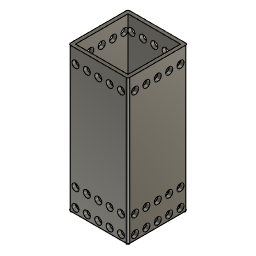
airbee_base (Autodesk Fusion 360 design; units mm, degrees)
Autodesk Fusion 360 part; units mm, degrees
sketch "Skizze1" plane through (0, 0, 0) normal (0, 0, 1) x (1, 0, 0)
  line L0 (-15, 15) -> (15, 15)
  line L1 (15, 15) -> (15, -15)
  line L2 (15, -15) -> (-15, -15)
  line L3 (-15, -15) -> (-15, 15)
  line L4 (17, -17) -> (-17, -17)
  line L5 (-17, -17) -> (-17, 17)
  line L6 (-17, 17) -> (17, 17)
  line L7 (17, 17) -> (17, -17)
  circle A0 centre (-10.16, 6.35) radius 3.5
  circle A1 centre (10.16, 6.35) radius 3.5
  circle A2 centre (-10.16, -6.35) radius 3.5
  circle A3 centre (10.16, -6.35) radius 3.5
  circle A4 centre (-10.16, 6.35) radius 0.75
  circle A5 centre (10.16, 6.35) radius 0.75
  circle A6 centre (10.16, -6.35) radius 0.75
  circle A7 centre (-10.16, -6.35) radius 0.75
  line L8 (-15, 3.5) -> (15, 3.5)
  line L9 (15, 3.5) -> (15, -3.5)
  line L10 (15, -3.5) -> (-15, -3.5)
  line L11 (-15, -3.5) -> (-15, 3.5)
  dimension "d3" = 30
  dimension "d4" = 30
  dimension "d5" = 15
  dimension "d6" = 15
  dimension "d7" = -2
  dimension "d8" = 7
  dimension "d9" = 7
  dimension "d10" = 7
  dimension "d11" = 7
  dimension "d12" = 20.32
  dimension "d16" = 4.84
  dimension "d19" = 4.84
  dimension "d20" = 12.7
  dimension "d21" = 20.32
  dimension "d22" = 12.7
  dimension "d23" = 8.65
  dimension "d25" = 8.65
  dimension "d26" = 1.5
  dimension "d27" = 1.5
  dimension "d28" = 1.5
  dimension "d29" = 1.5
  dimension "d140" = 7
  dimension "d141" = 3.5
  constraint horizontal L0
  constraint vertical L1
  constraint horizontal L2
  constraint vertical L3
  constraint concentric A0 A4
  constraint concentric A1 A5
  constraint concentric A3 A6
  constraint concentric A2 A7
  constraint horizontal L8
  constraint vertical L9
  constraint horizontal L10
  constraint vertical L11
  constraint coincident L1 L9.end
  constraint coincident L3 L8.start
  measures "d3" distance of L0.start L0.end
  measures "d4" distance of L0.start L2.end
  measures "d5" distance of origin L1
  measures "d6" distance of origin L2
  measures "d8" diameter of A0
  measures "d9" diameter of A1
  measures "d10" diameter of A3
  measures "d11" diameter of A2
  measures "d12" horizontal distance of A0.centre A1.centre
  measures "d16" distance of L3 A0.centre
  measures "d19" distance of L1 A3.centre
  measures "d20" distance of A1.centre A3.centre
  measures "d21" distance of A2.centre A3.centre
  measures "d22" vertical distance of A0.centre A2.centre
  measures "d23" distance of L0 A0.centre
  measures "d25" distance of L0 A1.centre
  measures "d26" diameter of A4
  measures "d27" diameter of A5
  measures "d28" diameter of A6
  measures "d29" diameter of A7
  measures "d140" distance of L8 L10
  measures "d141" distance of origin L8
extrude "Extrusion1" add sketch "Skizze1" against normal blind 2 contours L0 L1 L3 A0 A1 L8 | L1 L3 A0 A1 A2 A3 L8 L9 L10 L11 | L1 L2 L3 A2 A3 L10 | A0 L8 | A0 L8 | A1 L8 | A1 L8 | A2 L10 | A2 L10 | A3 L10 | A3 L10 | L4 L5 L6 L7 | A4 | A5 | A6 | A7
extrude "Extrusion2" add sketch "Skizze1" along normal blind 81 contours L4 L5 L6 L7
sketch "Skizze10" plane through (17, 0, 0) normal (1, 0, 0) x (0, 1, 0)
  line L0 (-15, 0) -> (15, 0)
  circle A0 centre (13, 2) radius 2
  circle A1 centre (6.5, 2) radius 2
  circle A2 centre (0, 2) radius 2
  circle A3 centre (-6.5, 2) radius 2
  circle A4 centre (-13, 2) radius 2
  circle A5 centre (13, 12.1429) radius 2
  circle A6 centre (6.5, 12.1429) radius 2
  circle A7 centre (0, 12.1429) radius 2
  circle A8 centre (-6.5, 12.1429) radius 2
  circle A9 centre (-13, 12.1429) radius 2
  circle A10 centre (13, 22.2857) radius 2
  circle A11 centre (6.5, 22.2857) radius 2
  circle A12 centre (0, 22.2857) radius 2
  circle A13 centre (-6.5, 22.2857) radius 2
  circle A14 centre (-13, 22.2857) radius 2
  circle A15 centre (13, 32.4286) radius 2
  circle A16 centre (6.5, 32.4286) radius 2
  circle A17 centre (0, 32.4286) radius 2
  circle A18 centre (-6.5, 32.4286) radius 2
  circle A19 centre (-13, 32.4286) radius 2
  circle A20 centre (13, 42.5714) radius 2
  circle A21 centre (6.5, 42.5714) radius 2
  circle A22 centre (0, 42.5714) radius 2
  circle A23 centre (-6.5, 42.5714) radius 2
  circle A24 centre (-13, 42.5714) radius 2
  circle A25 centre (13, 52.7143) radius 2
  circle A26 centre (6.5, 52.7143) radius 2
  circle A27 centre (0, 52.7143) radius 2
  circle A28 centre (-6.5, 52.7143) radius 2
  circle A29 centre (-13, 52.7143) radius 2
  circle A30 centre (13, 62.8571) radius 2
  circle A31 centre (6.5, 62.8571) radius 2
  circle A32 centre (0, 62.8571) radius 2
  circle A33 centre (-6.5, 62.8571) radius 2
  circle A34 centre (-13, 62.8571) radius 2
  circle A35 centre (13, 73) radius 2
  circle A36 centre (6.5, 73) radius 2
  circle A37 centre (0, 73) radius 2
  circle A38 centre (-6.5, 73) radius 2
  circle A39 centre (-13, 73) radius 2
  line L1 (-17, 81) -> (-17, -2)
  line L2 (-17, -2) -> (17, -2)
  line L3 (17, -2) -> (17, 81)
  line L4 (17, 81) -> (-17, 81)
  line L5 (15, 10) -> (-15, 10)
  line L6 (-15, 10) -> (-15, 81)
  line L7 (-15, 81) -> (15, 81)
  line L8 (15, 81) -> (15, 10)
  line L9 (15, 10) -> (-15, 10)
  line L10 (-15, 10) -> (-15, 6)
  line L11 (-15, 6) -> (15, 6)
  line L12 (15, 6) -> (15, 10)
  line L13 (15, 0) -> (15, 81)
  dimension "d146" = 4
  dimension "d151" = -26
  dimension "d152" = 71
  dimension "d197" = 2
  dimension "d198" = 2
  dimension "d199" = 71
  dimension "d200" = 4
  dimension "d201" = 2
  dimension "d202" = 2
  constraint horizontal L5
  constraint vertical L6
  constraint horizontal L7
  constraint vertical L8
  constraint coincident L4 L6.end
  constraint horizontal L9
  constraint vertical L10
  constraint horizontal L11
  constraint vertical L12
  measures "d146" diameter of A0
  measures "d197" distance of L3 L8
  measures "d198" distance of L1 L6
  measures "d199" distance of L5 L7
  measures "d200" distance of L5.start L11.end
  measures "d201" distance of L0 A0.centre
  measures "d202" distance of A0.centre L13
sketch "Skizze16" plane through (0, 17, 0) normal (0, 1, 0) x (-1, 0, 0)
  line L0 (-17, 81) -> (-17, -2)
  line L1 (-17, -2) -> (17, -2)
  line L2 (17, -2) -> (17, 81)
  line L3 (17, 81) -> (-17, 81)
  line L4 (-17, 81) -> (-17, -2)
  circle A0 centre (0, 52.7143) radius 2
  circle A1 centre (-6.5, 22.2857) radius 2
  circle A2 centre (13, 62.8571) radius 2
  circle A3 centre (6.5, 52.7143) radius 2
  line L5 (15, 6) -> (15, 10)
  circle A4 centre (0, 62.8571) radius 2
  circle A5 centre (6.5, 42.5714) radius 2
  circle A6 centre (-6.5, 62.8571) radius 2
  line L6 (-15, 0) -> (15, 0)
  circle A7 centre (13, 42.5714) radius 2
  circle A8 centre (13, 22.2857) radius 2
  circle A9 centre (-6.5, 2) radius 2
  circle A10 centre (6.5, 2) radius 2
  circle A11 centre (-6.5, 73) radius 2
  circle A12 centre (-13, 2) radius 2
  circle A13 centre (13, 73) radius 2
  circle A14 centre (6.5, 73) radius 2
  circle A15 centre (-13, 42.5714) radius 2
  circle A16 centre (13, 2) radius 2
  circle A17 centre (-6.5, 42.5714) radius 2
  line L7 (15, 0) -> (15, 81)
  circle A18 centre (-6.5, 52.7143) radius 2
  circle A19 centre (6.5, 32.4286) radius 2
  circle A20 centre (6.5, 62.8571) radius 2
  circle A21 centre (6.5, 12.1429) radius 2
  circle A22 centre (13, 52.7143) radius 2
  line L8 (15, 10) -> (-15, 10)
  circle A23 centre (-13, 12.1429) radius 2
  circle A24 centre (0, 2) radius 2
  circle A25 centre (-6.5, 12.1429) radius 2
  circle A26 centre (-13, 73) radius 2
  line L9 (-15, 81) -> (15, 81)
  line L10 (17, 81) -> (-17, 81)
  line L11 (-17, -2) -> (17, -2)
  circle A27 centre (13, 12.1429) radius 2
  circle A28 centre (0, 73) radius 2
  circle A29 centre (0, 12.1429) radius 2
  line L12 (-15, 6) -> (15, 6)
  circle A30 centre (13, 32.4286) radius 2
  line L13 (15, 10) -> (-15, 10)
  line L14 (-15, 10) -> (-15, 6)
  circle A31 centre (-6.5, 32.4286) radius 2
  circle A32 centre (-13, 62.8571) radius 2
  circle A33 centre (0, 22.2857) radius 2
  circle A34 centre (6.5, 22.2857) radius 2
  circle A35 centre (-13, 22.2857) radius 2
  circle A36 centre (0, 32.4286) radius 2
  circle A37 centre (-13, 32.4286) radius 2
  circle A38 centre (-13, 52.7143) radius 2
  line L15 (15, 81) -> (15, 10)
  line L16 (17, -2) -> (17, 81)
  line L17 (-15, 10) -> (-15, 81)
  circle A39 centre (0, 42.5714) radius 2
  dimension "d205" = -26
  dimension "d206" = 71
  dimension "d207" = 4
  dimension "d208" = 2
  dimension "d209" = 2
  dimension "d210" = 71
  dimension "d211" = 4
  dimension "d212" = 2
  dimension "d213" = 2
  constraint horizontal L13
  constraint vertical L17
  constraint horizontal L9
  constraint vertical L15
  constraint coincident L9.start L10
  constraint horizontal L8
  constraint vertical L14
  constraint horizontal L12
  constraint vertical L5
  measures "d207" diameter of A16
  measures "d208" distance of L15 L16
  measures "d209" distance of L4 L17
  measures "d210" distance of L9 L13
  measures "d211" distance of L5.start L5.end
  measures "d212" distance of A16.centre L6
  measures "d213" distance of A16.centre L7
sketch "Skizze17" plane through (-17, 0, 0) normal (-1, 0, 0) x (0, -1, 0)
  line L0 (-17, 81) -> (-17, -2)
  line L1 (-17, -2) -> (17, -2)
  line L2 (17, -2) -> (17, 81)
  line L3 (17, 81) -> (-17, 81)
  line L4 (-17, 81) -> (-17, -2)
  circle A0 centre (0, 52.7143) radius 2
  circle A1 centre (-6.5, 22.2857) radius 2
  circle A2 centre (13, 62.8571) radius 2
  circle A3 centre (6.5, 52.7143) radius 2
  line L5 (15, 6) -> (15, 10)
  circle A4 centre (0, 62.8571) radius 2
  circle A5 centre (6.5, 42.5714) radius 2
  circle A6 centre (-6.5, 62.8571) radius 2
  line L6 (-15, 0) -> (15, 0)
  circle A7 centre (13, 42.5714) radius 2
  circle A8 centre (13, 22.2857) radius 2
  circle A9 centre (-6.5, 2) radius 2
  circle A10 centre (6.5, 2) radius 2
  circle A11 centre (-6.5, 73) radius 2
  circle A12 centre (-13, 2) radius 2
  circle A13 centre (13, 73) radius 2
  circle A14 centre (6.5, 73) radius 2
  circle A15 centre (-13, 42.5714) radius 2
  circle A16 centre (13, 2) radius 2
  circle A17 centre (-6.5, 42.5714) radius 2
  line L7 (15, 0) -> (15, 81)
  circle A18 centre (-6.5, 52.7143) radius 2
  circle A19 centre (6.5, 32.4286) radius 2
  circle A20 centre (6.5, 62.8571) radius 2
  circle A21 centre (6.5, 12.1429) radius 2
  circle A22 centre (13, 52.7143) radius 2
  line L8 (15, 10) -> (-15, 10)
  circle A23 centre (-13, 12.1429) radius 2
  circle A24 centre (0, 2) radius 2
  circle A25 centre (-6.5, 12.1429) radius 2
  circle A26 centre (-13, 73) radius 2
  line L9 (-15, 81) -> (15, 81)
  line L10 (17, 81) -> (-17, 81)
  line L11 (-17, -2) -> (17, -2)
  circle A27 centre (13, 12.1429) radius 2
  circle A28 centre (0, 73) radius 2
  circle A29 centre (0, 12.1429) radius 2
  line L12 (-15, 6) -> (15, 6)
  circle A30 centre (13, 32.4286) radius 2
  line L13 (15, 10) -> (-15, 10)
  line L14 (-15, 10) -> (-15, 6)
  circle A31 centre (-6.5, 32.4286) radius 2
  circle A32 centre (-13, 62.8571) radius 2
  circle A33 centre (0, 22.2857) radius 2
  circle A34 centre (6.5, 22.2857) radius 2
  circle A35 centre (-13, 22.2857) radius 2
  circle A36 centre (0, 32.4286) radius 2
  circle A37 centre (-13, 32.4286) radius 2
  circle A38 centre (-13, 52.7143) radius 2
  line L15 (15, 81) -> (15, 10)
  line L16 (17, -2) -> (17, 81)
  line L17 (-15, 10) -> (-15, 81)
  circle A39 centre (0, 42.5714) radius 2
  dimension "d216" = -26
  dimension "d217" = 71
  dimension "d218" = 4
  dimension "d219" = 2
  dimension "d220" = 2
  dimension "d221" = 71
  dimension "d222" = 4
  dimension "d223" = 2
  dimension "d224" = 2
  constraint horizontal L13
  constraint vertical L17
  constraint horizontal L9
  constraint vertical L15
  constraint coincident L9.start L10
  constraint horizontal L8
  constraint vertical L14
  constraint horizontal L12
  constraint vertical L5
  measures "d218" diameter of A16
  measures "d219" distance of L15 L16
  measures "d220" distance of L4 L17
  measures "d221" distance of L9 L13
  measures "d222" distance of L5.start L5.end
  measures "d223" distance of A16.centre L6
  measures "d224" distance of A16.centre L7
sketch "Skizze18" plane through (0, -17, 0) normal (0, -1, 0) x (1, 0, 0)
  line L0 (-17, 81) -> (-17, -2)
  line L1 (-17, -2) -> (17, -2)
  line L2 (17, -2) -> (17, 81)
  line L3 (17, 81) -> (-17, 81)
  line L4 (-17, 81) -> (-17, -2)
  circle A0 centre (0, 52.7143) radius 2
  circle A1 centre (-6.5, 22.2857) radius 2
  circle A2 centre (13, 62.8571) radius 2
  circle A3 centre (6.5, 52.7143) radius 2
  line L5 (15, 6) -> (15, 10)
  circle A4 centre (0, 62.8571) radius 2
  circle A5 centre (6.5, 42.5714) radius 2
  circle A6 centre (-6.5, 62.8571) radius 2
  line L6 (-15, 0) -> (15, 0)
  circle A7 centre (13, 42.5714) radius 2
  circle A8 centre (13, 22.2857) radius 2
  circle A9 centre (-6.5, 2) radius 2
  circle A10 centre (6.5, 2) radius 2
  circle A11 centre (-6.5, 73) radius 2
  circle A12 centre (-13, 2) radius 2
  circle A13 centre (13, 73) radius 2
  circle A14 centre (6.5, 73) radius 2
  circle A15 centre (-13, 42.5714) radius 2
  circle A16 centre (13, 2) radius 2
  circle A17 centre (-6.5, 42.5714) radius 2
  line L7 (15, 0) -> (15, 81)
  circle A18 centre (-6.5, 52.7143) radius 2
  circle A19 centre (6.5, 32.4286) radius 2
  circle A20 centre (6.5, 62.8571) radius 2
  circle A21 centre (6.5, 12.1429) radius 2
  circle A22 centre (13, 52.7143) radius 2
  line L8 (15, 10) -> (-15, 10)
  circle A23 centre (-13, 12.1429) radius 2
  circle A24 centre (0, 2) radius 2
  circle A25 centre (-6.5, 12.1429) radius 2
  circle A26 centre (-13, 73) radius 2
  line L9 (-15, 81) -> (15, 81)
  line L10 (17, 81) -> (-17, 81)
  line L11 (-17, -2) -> (17, -2)
  circle A27 centre (13, 12.1429) radius 2
  circle A28 centre (0, 73) radius 2
  circle A29 centre (0, 12.1429) radius 2
  line L12 (-15, 6) -> (15, 6)
  circle A30 centre (13, 32.4286) radius 2
  line L13 (15, 10) -> (-15, 10)
  line L14 (-15, 10) -> (-15, 6)
  circle A31 centre (-6.5, 32.4286) radius 2
  circle A32 centre (-13, 62.8571) radius 2
  circle A33 centre (0, 22.2857) radius 2
  circle A34 centre (6.5, 22.2857) radius 2
  circle A35 centre (-13, 22.2857) radius 2
  circle A36 centre (0, 32.4286) radius 2
  circle A37 centre (-13, 32.4286) radius 2
  circle A38 centre (-13, 52.7143) radius 2
  line L15 (15, 81) -> (15, 10)
  line L16 (17, -2) -> (17, 81)
  line L17 (-15, 10) -> (-15, 81)
  circle A39 centre (0, 42.5714) radius 2
  dimension "d227" = -26
  dimension "d228" = 71
  dimension "d229" = 4
  dimension "d230" = 2
  dimension "d231" = 2
  dimension "d232" = 71
  dimension "d233" = 4
  dimension "d234" = 2
  dimension "d235" = 2
  constraint horizontal L13
  constraint vertical L17
  constraint horizontal L9
  constraint vertical L15
  constraint coincident L9.start L10
  constraint horizontal L8
  constraint vertical L14
  constraint horizontal L12
  constraint vertical L5
  measures "d229" diameter of A16
  measures "d230" distance of L15 L16
  measures "d231" distance of L4 L17
  measures "d232" distance of L9 L13
  measures "d233" distance of L5.start L5.end
  measures "d234" distance of A16.centre L6
  measures "d235" distance of A16.centre L7
extrude "Extrusion13" cut sketch "Skizze16" against normal blind 2 contours A26 | A23 | A27 | A13 | A16 | A9 | A10 | A11 | A12 | A14 | A21 | A24 | A25 | A28 | A29
extrude "Extrusion14" cut sketch "Skizze10" against normal blind 2 contours A0 | A1 | A2 | A3 | A4 | A5 | A35 | A39 | A9 | A6 | A7 | A8 | A36 | A37 | A38
extrude "Extrusion15" cut sketch "Skizze18" against normal blind 2 contours A26 | A23 | A27 | A13 | A16 | A9 | A10 | A11 | A12 | A14 | A21 | A24 | A25 | A28 | A29
extrude "Extrusion16" cut sketch "Skizze17" against normal blind 2 contours A26 | A23 | A27 | A13 | A16 | A9 | A10 | A11 | A12 | A14 | A21 | A24 | A25 | A28 | A29
fillet "Abrundung3" radius 1 8 edges at (17, 17, 39.5) (0, 17, -2) (17, 0, -2) (0, -17, -2) (-17, 0, -2) (-17, -17, 39.5) (17, -17, 39.5) (-17, 17, 39.5)
equation "d16 = ( 30 mm - 0.8 in ) / 2"
equation "d19 = ( 30 mm - 0.8 in ) / 2"
equation "d23 = ( 30 mm - 0.5 in ) / 2"
equation "d25 = ( 30 mm - 0.5 in ) / 2"
